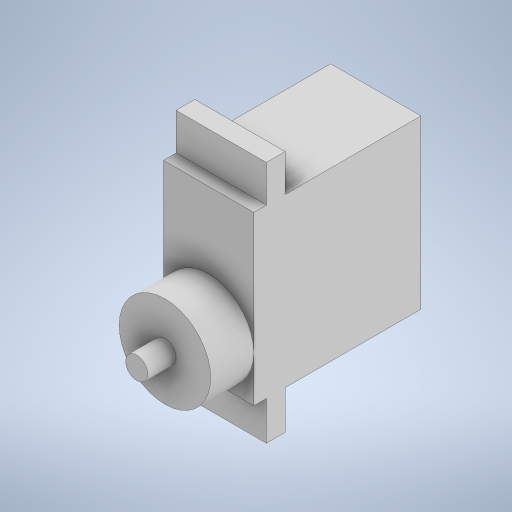
# Autodesk Inventor part: small servo
Saved by Autodesk Inventor 2024 (Build 280153000, 153)
## iProperties
Created: 2024-03-02
Part Number: small servo
Material: Generic
Document SubType Name: Modeling
Designer: dustp
Density: 1 g/cm^3
Appearance: Default
Author: dustp
Autodesk Inventor part; units mm, degrees
ref_plane "YZ Plane" through (0, 0, 0) normal (1, 0, 0) x (0, 1, 0)
ref_plane "XZ Plane" through (0, 0, 0) normal (0, 1, 0) x (-1, 0, 0)
ref_plane "XY Plane" through (0, 0, 0) normal (0, 0, 1) x (1, 0, 0)
sketch "Sketch1" plane through (0, 0, 0) normal (0, 0, 1) x (1, 0, 0)
  line L0 (0, 0) -> (12.192, 0)
  line L1 (12.192, 0) -> (12.192, 22.606)
  line L2 (12.192, 22.606) -> (0, 22.606)
  line L3 (0, 22.606) -> (0, 0)
  dimension "d0" = 12.192
  dimension "d1" = 22.606
  constraints: 8 end point, 2 parallel, 1 horizontal, 1 perpendicular
  measures "d0" distance of L2.end L1.end
  measures "d1" distance of L0.end L1.end
extrude "Extrusion1" add sketch "Sketch1" against normal blind 22.5552
sketch "Sketch2" plane through (0, 22.606, 0) normal (0, 1, 0) x (1, 0, 0)
  line L0 (12.192, 0) -> (12.192, 22.5552) projected
  line L1 (0, 1.6764) -> (12.192, 1.6764)
  line L2 (12.192, 1.6764) -> (12.192, 4.2164)
  line L3 (12.192, 4.2164) -> (0, 4.2164)
  line L4 (0, 4.2164) -> (0, 1.6764)
  line L5 (12.192, 0) -> (0, 0) projected
  dimension "d4" = 2.54
  dimension "d5" = 1.6764
  dimension "d6" = 4.2164
  constraints: 8 end point, 2 parallel, 1 horizontal, 1 perpendicular, 1 point on line
  measures "d4" distance of L2.end L1.end
  measures "d5" distance between parallel lines of L5 L1
  measures "d6" distance between parallel lines of L5 L3
extrude "Extrusion2" add sketch "Sketch2" along normal blind 5 and the other way blind 27.83
sketch "Sketch3" plane through (0, 0, 0) normal (0, 0, 1) x (1, 0, 0)
  circle A0 centre (6.02, 6.172) radius 6.172
  line L0 (12.192, 0) -> (12.192, 22.606) projected
  line L1 (0, 22.606) -> (0, 0) projected
  line L2 (0, 0) -> (12.192, 0) projected
  dimension "d11" = 6.172
  dimension "d12" = 12.192
  dimension "d13" = 6.02
  dimension "d14" = 12.344
  constraints: 2 tangent, 1 centre point
  measures "d11" distance from line of L0 A0.centre
  measures "d12" distance between parallel lines of L1 L0
  measures "d13" distance from line of L1 A0.centre
  measures "d14" diameter of A0
extrude "Extrusion3" add sketch "Sketch3" along normal blind 5.842 contours A0 L1 | L1 A0
sketch "Sketch4" plane through (6.02, 6.172, 5.842) normal (0, 0, 1) x (1, 0, 0)
  circle A0 centre (0, 0) radius 1.5
  line L0 (0, -6.172) -> (6.172, -6.172) projected
  line L1 (6.172, 16.434) -> (-6.02, 16.434) projected
  line L2 (-6.02, 16.434) -> (-6.02, 1.3613) projected
  line L3 (6.172, 0) -> (6.172, 16.434) projected
  point P0 (-6.02, -6.172)
  dimension "d17" = 3
  dimension "d24" = 22.606
  dimension "d25" = 12.192
  constraints: 1 centre point
  measures "d17" diameter of A0
  measures "d24" distance between parallel lines of L0 L1
  measures "d25" distance between parallel lines of L2 L3
extrude "Extrusion4" add sketch "Sketch4" along normal blind 3.81
body "Solid1"
